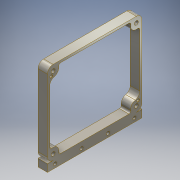
# Autodesk Inventor part: Корпус03
Saved by Autodesk Inventor 2016 (Build 200138000, 138)
## iProperties
Created: 2021-04-23
Part Number: Корпус03
Material: Типовые
Document SubType Name: Modeling
Designer: Лол
Density: 1 g/cm^3
Appearance: Титан — полированный
Author: Лол
Autodesk Inventor part; units mm, degrees
ref_plane "YZ Plane" through (0, 0, 0) normal (1, 0, 0) x (0, 1, 0)
ref_plane "XZ Plane" through (0, 0, 0) normal (0, 1, 0) x (-1, 0, 0)
ref_plane "XY Plane" through (0, 0, 0) normal (0, 0, 1) x (1, 0, 0)
sketch "Эскиз1" plane through (0, 0, 0) normal (0, 0, 1) x (1, 0, 0)
  line L0 (-12.5, 120) -> (12.5, 120)
  line L1 (12.5, 120) -> (12.5, -130)
  line L2 (12.5, -130) -> (-12.5, -130)
  line L3 (-12.5, -130) -> (-12.5, 120)
  line L4 (-17.5, 0) -> (17.5, 0) projected
  line L5 (0, -180) -> (0, 170) projected
  point P0 (0, 0)
  dimension "d0" = 250
  dimension "d1" = 25
  dimension "d2" = 120
  constraints: 8 end point, 2 parallel, 1 horizontal, 1 perpendicular, 1 other
  measures "d0" distance of L0.end L1.end
  measures "d1" distance of L0.start L0.end
  measures "d2" distance between parallel lines of L4 L0
extrude "Выдавливание1" add sketch "Эскиз1" along normal blind 100 and the other way blind 120
sketch "Эскиз2" plane through (12.5, -130, 100) normal (1, 0, 0) x (0, 0, -1)
  line L0 (0, 250) -> (220, 250) projected
  line L1 (0, 0) -> (0, 250) projected
  line L2 (220, 250) -> (220, 0) projected
  line L3 (0, 0) -> (220, 0) projected
  line L4 (6, 244) -> (214, 244)
  line L5 (214, 244) -> (214, 6)
  line L6 (214, 6) -> (6, 6)
  line L7 (6, 6) -> (6, 244)
  point P0 (100, 130)
  dimension "d7" = 6
  dimension "d8" = 6
  dimension "d9" = 6
  dimension "d10" = 6
  constraints: 8 end point, 2 parallel, 1 horizontal, 1 perpendicular
  measures "d7" distance between parallel lines of L0 L4
  measures "d8" distance between parallel lines of L2 L5
  measures "d9" distance between parallel lines of L3 L6
  measures "d10" distance between parallel lines of L1 L7
extrude "Выдавливание2" cut sketch "Эскиз2" against normal through all contours L4 L5 L6 L7
fillet "Сопряжение1" radius 15 4 edges at (0, 120, 100) (0, 120, -120) (0, -130, 100) (0, -130, -120)
sketch "Эскиз3" plane through (12.5, -115, -120) normal (1, 0, 0) x (0, 0, -1)
  arc A0 (-205, 235) -> (-220, 220) centre (-205, 220) ccw projected
  arc A1 (0, 220) -> (-15, 235) centre (-15, 220) ccw projected
  arc A2 (-15, -15) -> (0, 0) centre (-15, 0) ccw projected
  arc A3 (-220, 0) -> (-205, -15) centre (-205, 0) ccw projected
  arc A4 (-15, -15) -> (0, 0) centre (-15, 0) ccw projected
  circle A5 centre (-205, 0) radius 15
  circle A6 centre (-15, 0) radius 15
  circle A7 centre (-15, 220) radius 15
  circle A8 centre (-205, 220) radius 15
  point P0 (-120, 115)
  dimension "d15" = 30
  constraints: 4 centre point, 4 coincident, 3 equal radius
  measures "d15" diameter of A8
extrude "Выдавливание3" add sketch "Эскиз3" against normal up to surface (25 mm away)
fillet "Сопряжение2" radius 5 6 edges at (0, 93, 94) (0, 93, -114) (0, -103, -114) (0, -103, 94) (0, 114, 73) (0, -124, -93)
sketch "Эскиз4" plane through (-12.5, -115, -120) normal (-1, 0, 0) x (0, 0, 1)
  line L0 (0, 0) -> (0, 220) projected
  arc A0 (0, 0) -> (15, -15) centre (15, 0) ccw projected
  line L1 (205, -15) -> (15, -15) projected
  arc A1 (205, -15) -> (220, 0) centre (205, 0) ccw projected
  line L2 (220, 220) -> (220, 0) projected
  arc A2 (220, 220) -> (205, 235) centre (205, 220) ccw projected
  line L3 (15, 235) -> (205, 235) projected
  arc A3 (15, 235) -> (0, 220) centre (15, 220) ccw projected
  line L4 (27, 229) -> (185.4041, 229) projected
  arc A4 (190.3031, 223) -> (208, 205.3031) centre (205, 220) ccw projected
  arc A5 (214, 200.4041) -> (208, 205.3031) centre (209, 200.4041) ccw projected
  line L5 (214, 200.4041) -> (214, 19.5959) projected
  arc A6 (208, 14.6969) -> (214, 19.5959) centre (209, 19.5959) ccw projected
  arc A7 (208, 14.6969) -> (193, -9) centre (205, 0) ccw projected
  line L6 (193, -9) -> (34.5959, -9) projected
  arc A8 (29.6969, -3) -> (12, 14.6969) centre (15, 0) ccw projected
  arc A9 (6, 19.5959) -> (12, 14.6969) centre (11, 19.5959) ccw projected
  line L7 (6, 19.5959) -> (6, 200.4041) projected
  arc A10 (12, 205.3031) -> (6, 200.4041) centre (11, 200.4041) ccw projected
  arc A11 (12, 205.3031) -> (27, 229) centre (15, 220) ccw projected
  circle A12 centre (15, 0) radius 5.1
  circle A13 centre (15, 220) radius 5.1
  arc A14 (220, 220) -> (205, 235) centre (205, 220) ccw projected
  circle A15 centre (205, 220) radius 5.1
  circle A16 centre (205, 0) radius 5.1
  arc A17 (190.3031, 223) -> (185.4041, 229) centre (185.4041, 224) ccw projected
  arc A18 (29.6969, -3) -> (34.5959, -9) centre (34.5959, -4) ccw projected
  point P0 (120, 115)
  dimension "d19" = 10.2
  constraints: 4 centre point, 4 coincident, 3 equal radius
  measures "d19" diameter of A12
extrude "Выдавливание4" cut sketch "Эскиз4" against normal through all contours A12 | A13 | A15 | A16
fillet "Сопряжение4" radius 15 2 edges at (0, 114, -93) (0, -124, 73)
sketch "Эскиз6" plane through (-12.5, -115, -120) normal (-1, 0, 0) x (0, 0, 1)
  circle A0 centre (15, 220) radius 5.1 projected
  circle A1 centre (205, 0) radius 5.1 projected
  circle A2 centre (195, -5) radius 3
  circle A3 centre (25, 225) radius 3
  point P0 (120, 115)
  dimension "d35" = 6
  dimension "d37" = 10
  dimension "d38" = 5
  dimension "d39" = 230
  dimension "d40" = 170
  constraints: 2 centre point, 1 equal radius
  measures "d35" diameter of A3
  measures "d37" horizontal distance of A2.centre A1.centre
  measures "d38" vertical distance of A1.centre A2.centre
  measures "d39" vertical distance of A3.centre A2.centre
  measures "d40" horizontal distance of A3.centre A2.centre
extrude "Выдавливание6" cut sketch "Эскиз6" against normal through all contours A2 | A3
chamfer "Фаска2" distance 0.6 angle 45 4 edges at (-12.5, 110, -98) (-12.5, -120, 72) (12.5, -120, 72) (12.5, 110, -98)
sketch "Эскиз7" plane through (12.5, -115, 100) normal (1, 0, 0) x (0, 0, -1)
  line L0 (15, -15) -> (205, -15) projected
  line L1 (220, 220) -> (220, 0) projected
  line L2 (15, 235) -> (205, 235) projected
  line L3 (220, -15) -> (240, -15)
  line L4 (240, -15) -> (240, 235)
  line L5 (240, 235) -> (220, 235)
  line L6 (220, 235) -> (220, -15)
  line L7 (230, -15) -> (230, 235) construction
  circle A0 centre (230, 5) radius 4.25
  circle A1 centre (230, 75) radius 4.25
  circle A2 centre (230, 145) radius 4.25
  circle A3 centre (230, 215) radius 4.25
  point P0 (100, 115)
  dimension "d46" = 20
  dimension "d49" = 8.5
  dimension "d50" = 20
  dimension "d51" = 70
  dimension "d52" = 20
  dimension "d53" = 70
  constraints: 10 end point, 4 centre point, 4 collinear, 4 point on line, 3 equal radius, 2 midpoint, 2 parallel, 1 horizontal, 1 perpendicular
  measures "d46" distance of L4.end L5.end
  measures "d49" diameter of A0
  measures "d50" distance from line of A0.centre L3
  measures "d51" distance of A1.centre A0.centre
  measures "d52" distance from line of L5 A3.centre
  measures "d53" distance of A2.centre A3.centre
extrude "Выдавливание7" add sketch "Эскиз7" against normal up to surface (25 mm away) contours L6 L5 L4 L3 L1 | A0 | A1 | A2 | A3
extrude "Выдавливание8" cut sketch "Эскиз7" against normal through all contours A0 | A1 | A2 | A3
